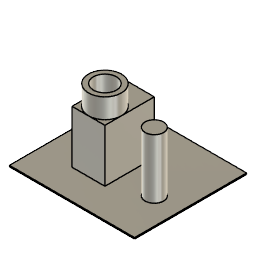
PIR Housing Recepticle (Autodesk Fusion 360 design; units mm, degrees)
Autodesk Fusion 360 part; units mm, degrees
sketch "Sketch1" plane through (0, 0, 0) normal (0, 0, 1) x (1, 0, 0)
  line L0 (0, 0) -> (5, 0)
  line L1 (5, 0) -> (5, -7.5)
  line L2 (5, -7.5) -> (0, -7.5)
  line L3 (0, -7.5) -> (0, 0)
  dimension "d1" = 5
  dimension "d2" = 7.5
  constraint horizontal L0
  constraint vertical L1
  constraint horizontal L2
  constraint vertical L3
  constraint coincident L0.start L3.end
  measures "d1" distance of L0.start L0.end
  measures "d2" distance of L0.start L2.end
extrude "Extrude1" add sketch "Sketch1" along normal blind 8 makes body 1
sketch "Sketch2" plane through (0, 0, 8) normal (0, 0, 1) x (-1, 0, 0)
  line L0 (0, 7.5) -> (-5, 7.5)
  line L1 (-5, 7.5) -> (-5, 0)
  line L2 (-5, 0) -> (0, 0)
  line L3 (0, 0) -> (0, 7.5)
  circle A0 centre (-2.5, 5) radius 2.5
  circle A1 centre (-2.5, 5) radius 1.75
  dimension "d5" = 3.5
  constraint tangent L1 A0
  constraint concentric A0 A1
  measures "d5" diameter of A1
extrude "Extrude2" add sketch "Sketch2" along normal blind 3 contours A0 bodies 1
sketch "Sketch3" plane through (0, 0, 0) normal (0, 0, 1) x (1, 0, 0)
  circle A0 centre (10, -5) radius 1.4
  dimension "d8" = 2.8
  measures "d8" diameter of A0
extrude "Extrude3" add sketch "Sketch3" along normal blind 9 separate body makes body 2
extrude "Extrude4" cut 1 faces at (2.4138, -5.3569, 8) along direction (0, 0, -1) blind 6 on bodies 1 bodies 1
sketch "Sketch4" plane through (0, 0, 0) normal (0, 0, -1) x (1, 0, 0)
  line L0 (5, 7.5) -> (0, 7.5)
  line L1 (0, 7.5) -> (0, 0)
  line L2 (0, 0) -> (5, 0)
  line L3 (5, 0) -> (5, 7.5)
  line L4 (-5, 12) -> (14, 12)
  line L5 (14, 12) -> (14, -5)
  line L6 (14, -5) -> (-5, -5)
  line L7 (-5, -5) -> (-5, 12)
  constraint horizontal L4
  constraint vertical L5
  constraint horizontal L6
  constraint vertical L7
extrude "Extrude5" add sketch "Sketch4" along normal blind 0.2 contours L0 L1 L2 L3 | L4 L5 L6 L7 bodies 1 2
